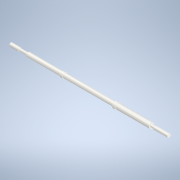
# Autodesk Inventor part: Eje
Saved by Autodesk Inventor 2020 (Build 240168000, 168)
## iProperties
CustomPartVersion: 1
Created: 2021-01-12
Part Number: Eje
Material: Steel
Document SubType Name: Modeling
Designer: User
Density: 1 g/cm^3
Appearance: Steel
Length: 875,000 mm
Author: User
Autodesk Inventor part; units mm, degrees
ref_plane "Plano inicial" through (0, 0, 0) normal (1, 0, 0) x (0, 1, 0)
ref_plane "XZ Plane" through (0, 0, 0) normal (0, 1, 0) x (-1, 0, 0)
ref_plane "XY Plane" through (0, 0, 0) normal (0, 0, 1) x (1, 0, 0)
sketch "Boceto principal" plane through (0, 0, 0) normal (0, 0, 1) x (1, 0, 0)
  line L0 (0, 0) -> (875, 0)
  line L1 (0, 0) -> (0, 10)
  line L2 (65, 7.5) -> (65, 12.5)
  line L3 (0, 10) -> (50, 10)
  line L4 (65, 12.5) -> (260, 12.5)
  line L5 (260, 12.5) -> (260, 15)
  line L6 (275, 15) -> (275, 12.5)
  line L7 (260, 15) -> (275, 15)
  line L8 (275, 12.5) -> (565, 12.5)
  line L9 (565, 12.5) -> (565, 17.5)
  line L10 (580, 17.5) -> (580, 15)
  line L11 (565, 17.5) -> (580, 17.5)
  line L12 (775, 15) -> (775, 7.5)
  line L13 (580, 15) -> (775, 15)
  line L14 (795, 7.5) -> (795, 10)
  line L15 (775, 7.5) -> (795, 7.5)
  line L16 (875, 10) -> (875, 0)
  line L17 (795, 10) -> (875, 10)
  line L18 (50, 10) -> (50, 7.5)
  line L19 (50, 7.5) -> (65, 7.5)
  dimension "d3" = 20
  dimension "d5" = 25
  dimension "d6" = 30
  dimension "d7" = 25
  dimension "d8" = 35
  dimension "d9" = 30
  dimension "d10" = 15
  dimension "d11" = 20
  dimension "d12" = 15
  constraints: 40 end point, 10 vertical, 1 horizontal
  measures "d3" diameter of L3 L0
  measures "d5" diameter of L4 L0
  measures "d6" diameter of L7 L0
  measures "d7" diameter of L8 L0
  measures "d8" diameter of L11 L0
  measures "d9" diameter of L13 L0
  measures "d10" diameter of L15 L0
  measures "d11" diameter of L17 L0
  measures "d12" diameter of L19 L0
revolve "Revolución1" add sketch "Boceto principal" angle 360 about axis through (0, 0, 0) along (1, 0, 0)
equation "\"Length\" = 875"
